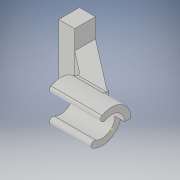
# Autodesk Inventor part: Roller_Spacer
Saved by Autodesk Inventor 2019 (Build 230136000, 136)
## iProperties
Created: 2019-10-12
Part Number: Roller_Spacer
Material: Generic
Document SubType Name: Modeling
Designer: James
Density: 1 g/cm^3
Appearance: Default
Author: James
Autodesk Inventor part; units mm, degrees
ref_plane "YZ Plane" through (0, 0, 0) normal (1, 0, 0) x (0, 1, 0)
sketch "Sketch1" plane through (0, 0, 0) normal (1, 0, 0) x (0, 1, 0)
  arc A0 (-3.4641, 2) -> (3.4641, 2) centre (0, 0) ccw
  arc A1 (-5.1962, 3) -> (5.1962, 3) centre (0, 0) ccw
  arc A2 (5.1962, 3) -> (3.4641, 2) centre (4.3301, 2.5) ccw
  arc A3 (-3.4641, 2) -> (-5.1962, 3) centre (-4.3301, 2.5) ccw
  dimension "d0" = 8
  dimension "d1" = 12
  dimension "d2" = 2.5
  constraints: 8 point on circle, 4 centre point, 3 tangent, 2 coincident, 1 equal radius, 1 horizontal alignment
  measures "d0" diameter of A0
  measures "d1" diameter of A1
  measures "d2" vertical distance of point (0, 0) A2.centre
extrude "Extrusion1" add sketch "Sketch1" along normal blind 16
sketch "Sketch4" plane through (16, 0, 0) normal (1, 0, 0) x (0, 0, -1)
  point P0 (0, 0)
sketch "Sketch5" plane through (16, 0, 0) normal (1, 0, 0) x (0, 0, -1)
  line L0 (-6.2503, -10.1933) -> (7.7655, -10.1933)
  line L1 (7.7655, -10.1933) -> (7.7655, 0)
  line L2 (7.7655, 0) -> (-6.2503, 0)
  line L3 (-6.2503, 0) -> (-6.2503, -10.1933)
  point P0 (0, 0)
  constraints: 8 end point, 2 parallel, 1 horizontal, 1 perpendicular
extrude "Extrusion4" cut sketch "Sketch5" against normal blind 3
ref_plane "Work Plane1" through (-7, 0, 0) normal (-1, 0, 0) x (0, 0, 1)
sketch "Sketch9" plane through (-7, 0, 0) normal (-1, 0, 0) x (0, 0, 1)
  line L0 (-17.9, 10) -> (-11.4, 10)
  line L1 (-11.4, 10) -> (-11.4, -10)
  line L2 (-11.4, -10) -> (-17.9, -10)
  line L3 (-17.9, -10) -> (-17.9, 10)
  point P0 (0, 0)
  point P1 (-17.9, 0)
  dimension "d34" = 11.4
  dimension "d35" = 6.5
  dimension "d36" = 20
  constraints: 8 end point, 2 parallel, 1 horizontal, 1 horizontal alignment, 1 midpoint, 1 perpendicular
  measures "d34" distance from line of point (0, 0) L1
  measures "d35" distance of L0.start L0.end
  measures "d36" distance of L2.end L0.start
extrude "Extrusion8" add sketch "Sketch9" along normal blind 5
ref_plane "Work Plane2" through (-7, 0, -17.9) normal (0, -1, 0) x (1, 0, 0)
sketch "Sketch10" plane through (-7, 0, -17.9) normal (0, -1, 0) x (1, 0, 0)
  line L0 (7, 11) -> (23, 11) projected
  line L1 (0, 0) -> (0, 6.5) projected
  line L2 (7, 11.9) -> (0, 6.5)
  line L3 (0, 0) -> (-5, 0) projected
  line L4 (0, 6.5) -> (0, 0)
  line L5 (0, 0) -> (15.4259, 11.9)
  line L6 (7, 11.9) -> (7, 20.9) projected
  line L7 (15.4259, 11.9) -> (7, 11.9)
  point P0 (7, 17.9)
  constraints: 8 end point, 2 perpendicular, 1 parallel, 2 other
extrude "Extrusion9" add sketch "Sketch10" along normal mid plane 8
sketch "Sketch11" plane through (0, 0, 0) normal (-1, 0, 0) x (0, 0, 1)
  line L0 (-6, -4) -> (-6, 0) projected
  line L1 (-6, -4) -> (-4.4721, -4)
  arc A0 (-6, 0) -> (3, -5.1962) centre (0, 0) ccw projected
  line L2 (-6, 4) -> (-6, 0) projected
  line L3 (-6, 4) -> (-4.4721, 4)
  arc A1 (3, 5.1962) -> (-6, 0) centre (0, 0) ccw projected
  constraints: 4 end point, 2 horizontal, 2 point on circle
extrude "Extrusion10" add sketch "Sketch11" against normal blind 9.1
fillet "Fillet3" radius 2 2 edges at (4.55, 4, -4.4721) (4.55, -4, -4.4721)
body "Solid1"
